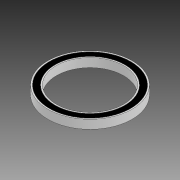
# Autodesk Inventor part: 6820 bearing
Saved by Autodesk Inventor 2020 (Build 240168000, 168)
## iProperties
Created: 2021-03-19
Part Number: 6820 bearing
Material: Generic
Document SubType Name: Modeling
Designer: DDeGo
Density: 1 g/cm^3
Appearance: Default
Author: DDeGo
Autodesk Inventor part; units mm, degrees
ref_plane "YZ Plane" through (0, 0, 0) normal (1, 0, 0) x (0, 1, 0)
ref_plane "XZ Plane" through (0, 0, 0) normal (0, 1, 0) x (-1, 0, 0)
ref_plane "XY Plane" through (0, 0, 0) normal (0, 0, 1) x (1, 0, 0)
sketch "Sketch1" plane through (0, 0, 0) normal (1, 0, 0) x (0, 1, 0)
  line L0 (0, 0) -> (13, 0) construction
  line L1 (13, 0) -> (13, -50) construction
  line L2 (13, -50) -> (0, -50)
  line L3 (0, -50) -> (0, 0) construction
  line L4 (13, -62.5) -> (0, -62.5)
  line L5 (13, -52) -> (12.8, -52)
  line L6 (12.8, -52) -> (12.8, -60.5)
  line L7 (12.8, -60.5) -> (13, -60.5)
  line L8 (0, -52) -> (0.2, -52)
  line L9 (0.2, -52) -> (0.2, -60.5)
  line L10 (0.2, -60.5) -> (0, -60.5)
  line L11 (13, -50) -> (13, -52)
  line L12 (13, -60.5) -> (13, -62.5)
  line L13 (0, -62.5) -> (0, -60.5)
  line L14 (0, -52) -> (0, -50)
  dimension "d0" = 50
  dimension "d2" = 13
  dimension "d5" = 62.5
  dimension "d6" = 0.2
  dimension "d7" = 2
  constraints: 30 end point, 7 perpendicular, 4 collinear, 4 point on line, 3 horizontal, 3 vertical
  measures "d0" distance between parallel lines of L0 L2
  measures "d2" distance of L0.start L0.end
  measures "d5" distance between parallel lines of L0 L4
  measures "d6" distance of L8.start L8.end
  measures "d7" distance of L8.start L2.end
revolve "Revolution1" add sketch "Sketch1" angle 360 about axis through (0, 0, 0) along (0, 1, 0)
body "Solid1"
